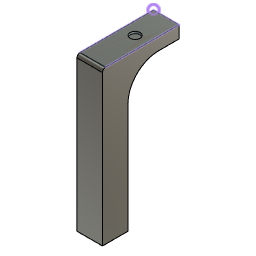
stand (Autodesk Fusion 360 design; units mm, degrees)
Autodesk Fusion 360 part; units mm, degrees
note: some values were not read from the file. Chosen so that the rebuilt part matches the saved one: which face or edge a step refers to.
sketch "Esquisse1" plane through (0, 0, 0) normal (1, 0, 0) x (0, 1, 0)
  line L0 (0, 0) -> (25, 0)
  line L1 (25, 0) -> (25, 25)
  line L2 (25, 25) -> (0, 25)
  line L3 (0, 25) -> (0, 0)
  dimension "d1" = 25
  dimension "d2" = 25
  constraint horizontal L0
  constraint vertical L1
  constraint horizontal L2
  constraint vertical L3
  constraint coincident L0.start L3.end
  measures "d1" distance of L0.start L0.end
  measures "d2" distance of L0.start L2.end
sketch "Esquisse2" plane through (0, 0, 0) normal (0, 0, 1) x (1, 0, 0)
  line L0 (0, 0) -> (-25, 0)
  line L1 (-25, 0) -> (-25, -25)
  line L2 (-25, -25) -> (0, -25)
  line L3 (0, -25) -> (0, 0)
  dimension "d5" = 25
  dimension "d6" = 25
  constraint horizontal L0
  constraint vertical L1
  constraint horizontal L2
  constraint vertical L3
  constraint coincident L0.start L3.end
  measures "d5" distance of L0.start L0.end
  measures "d6" distance of L0.start L2.end
extrude "Extrusion2" add sketch "Esquisse2" along normal blind 150
sketch "Esquisse3" plane through (0, 0, 0) normal (0, 0, 1) x (1, 0, 0)
ref_plane "Plan de construction1" through (0, 0, 0) normal (0, 1, 0) x (0, 0, 1)
sketch "Esquisse4" plane through (0, 0, 0) normal (0, 1, 0) x (1, 0, 0)
  line L0 (-25, -150) -> (0, -150)
  line L1 (0, -150) -> (0, -138)
  line L2 (0, -138) -> (-25, -138)
  line L3 (-25, -138) -> (-25, -150)
  dimension "d12" = 25
  dimension "d13" = 12
  constraint horizontal L0
  constraint vertical L1
  constraint horizontal L2
  constraint vertical L3
  measures "d12" distance of L0.start L0.end
  measures "d13" distance of L0.start L2.end
extrude "Extrusion3" add sketch "Esquisse4" along normal blind 50
fillet "Congé4" radius 3 1 edges at (-12.5, -25, 150)
sketch "Esquisse5" plane through (0, 0, 0) normal (0, 0, 1) x (1, 0, 0)
  arc A0 (-49.9758, 74.9967) -> (-29.9758, 49.9967) centre (-26.8195, 73.0218) ccw
  line L0 (-49.9758, 74.9967) -> (-45.791, 74.9967)
  line L1 (-29.9758, 54.2107) -> (-29.9758, 49.9967)
  arc A1 (-45.791, 74.9967) -> (-29.9758, 54.2107) centre (-26.8195, 73.0218) ccw
  constraint horizontal L0
  constraint vertical L1
  constraint concentric A0 A1
sketch "Esquisse6" plane through (0, 0, 0) normal (0, 0, -1) x (1, 0, 0)
  line L0 (-25, 0) -> (0, 0)
  line L1 (0, 0) -> (0, 25)
  line L2 (0, 25) -> (-25, 25)
  line L3 (-25, 25) -> (-25, 0)
  line L4 (-24.1213, 24.1213) -> (-0.8787, 0.8787) construction
  circle A0 centre (-3.6105, 3.6105) radius 2.25
  circle A1 centre (-20, 20) radius 2.25
  dimension "d28" = 4.5
  dimension "d29" = 4.5
  constraint coincident L4 A0.centre
  constraint coincident L4 A1.centre
  measures "d28" diameter of A1
  measures "d29" diameter of A0
extrude "Extrusion5" cut sketch "Esquisse6" against normal blind 22 contours A0 | A1
sketch "Esquisse7" plane through (0, 0, 150) normal (0, 0, 1) x (-1, 0, 0)
  line L0 (25, 22) -> (0, 22)
  line L1 (0, -50) -> (25, -50)
  line L2 (25, -50) -> (25, 22)
  line L3 (0, 22) -> (0, -50)
sketch "Esquisse8" plane through (0, 0, 150) normal (0, 0, 1) x (-1, 0, 0)
  line L0 (12.5, -50) -> (12.5, -46.968) construction
  line L1 (12.5, -46.968) -> (12.5, 8.032) construction
  line L2 (3, -50) -> (22, -50) construction
  circle A0 centre (12.5, -19.468) radius 4.9431
  dimension "d32" = 55
  constraint vertical L0
  constraint vertical L1
  constraint coincident L0.start L2
  constraint midpoint L0.start L2
  constraint midpoint L1 A0.centre
  measures "d32" distance of L0.end L1.end
extrude "Extrusion6" cut sketch "Esquisse8" against normal blind 2
fillet "Congé5" radius 30 1 edges at (-12.5, 0, 138)
